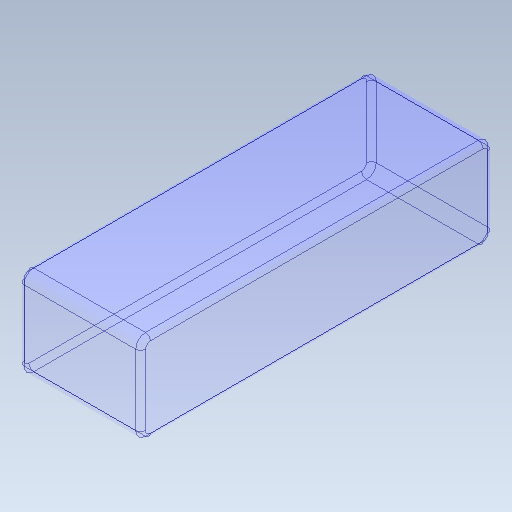
# Autodesk Inventor part: 4S5000
Saved by Autodesk Inventor 2020 (Build 240168000, 168)
## iProperties
Part Number: 4S5000
Material: ABS-Kunststoff
Document SubType Name: Modeling
Designer: Admin
Mass: 282.972 g
Surface Area: 279.425 cm^2
Volume: 266.955 cm^3
Density: 1.06 g/cm^3
Appearance: GEDA zusätzlich blau transp. A
Gewicht: 0,043 kg
G_L: 0
G_H: 0
G_B: 0
InventorVersion: 2019.4
VAULT_Status: in Bearbeitung
Revision: -
Max. Breite: 0
Max. Höhe: 0
Max. Länge: 0
Max. Abmessungen: 0 x 0 x 0
Author: Admin
Autodesk Inventor part; units mm, degrees
note: some values were not read from the file. Left out: dimensions or parameters whose unit could not be read.
ref_plane "YZ Plane" through (0, 0, 0) normal (1, 0, 0) x (0, 1, 0)
ref_plane "XZ Plane" through (0, 0, 0) normal (0, 1, 0) x (-1, 0, 0)
ref_plane "XY Plane" through (0, 0, 0) normal (0, 0, 1) x (1, 0, 0)
sketch "Skizze1" plane through (0, 0, 0) normal (0, 0, 1) x (1, 0, 0)
  line L0 (-25, -72.5) -> (25, -72.5)
  line L1 (25, -72.5) -> (25, 72.5)
  line L2 (25, 72.5) -> (-25, 72.5)
  line L3 (-25, 72.5) -> (-25, -72.5)
  line L4 (-25, -72.5) -> (25, 72.5) construction
  line L5 (25, -72.5) -> (-25, 72.5) construction
  point P0 (0, 0)
  dimension "d0" = 50
  dimension "d1" = 145
  constraints: 12 end point, 2 midpoint, 2 parallel, 1 horizontal, 1 perpendicular
  measures "d0" distance of L2.end L1.end
  measures "d1" distance of L1.end L0.end
extrude "Extrusion1" add sketch "Skizze1" along normal blind 37
fillet "Rundung1" radius 4 4 edges at (0, 72.5, 37) (0, 72.5, 0) (0, -72.5, 0) (0, -72.5, 37)
fillet "Rundung1" radius 2 8 edges at (25, 0, 37) (25, -72.5, 18.5) (-25, -72.5, 18.5) (-25, 0, 37) (25, 0, 0) (25, 72.5, 18.5) (-25, 72.5, 18.5) (-25, 0, 0)
equation "\"G_L\" = 0"
equation "\"G_H\" = 0"
equation "\"G_B\" = 0"
